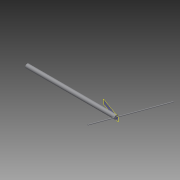
# Autodesk Inventor part: Piston_Model
Saved by Autodesk Inventor 2015 (Build 190159000, 159)
## iProperties
Created: 2017-01-24
Part Number: Piston_Model
Material: Generic
Document SubType Name: Modeling
Designer: Guy
Density: 1 g/cm^3
Appearance: Default
Author: Guy
Autodesk Inventor part; units mm, degrees
ref_plane "YZ Plane" through (0, 0, 0) normal (1, 0, 0) x (0, 1, 0)
ref_plane "XZ Plane" through (0, 0, 0) normal (0, 1, 0) x (-1, 0, 0)
ref_plane "XY Plane" through (0, 0, 0) normal (0, 0, 1) x (1, 0, 0)
sketch "Sketch1" plane through (0, 0, 0) normal (1, 0, 0) x (0, 1, 0)
  circle A0 centre (0, 0) radius 4.435
  dimension "d0" = 8.87
  constraints: 1 centre point, 1 coincident
  measures "d0" diameter of A0
extrude "Extrusion1" add sketch "Sketch1" along normal blind 200
sketch "Sketch2" plane through (200, 0, 0) normal (1, 0, 0) x (0, 0, -1)
  circle A0 centre (0, 0) radius 4.435 projected
  line L0 (0, 0) -> (8.3226, 0)
  line L1 (0.8914, 0) -> (-7.5966, 0)
  arc A1 (-4.435, 0) -> (4.435, 0) centre (0, 0) ccw
  constraints: 4 end point, 3 point on line, 2 horizontal, 2 point on circle, 1 centre point, 1 coincident, 1 concentric
extrude "Extrusion2" add sketch "Sketch2" along normal blind 0.01 contours A0 L1 L0 picked at (-2.4155, -1.6673)
ref_plane "Work Plane1" through (200.01, 0, 0) normal (0.3420201, 0.9396926, 0) x (0, 0, 1)
sketch "Sketch4" plane through (200.01, 0, 0) normal (0.3420201, 0.9396926, 0) x (0, 0, 1)
  line L0 (4.435, -0.0094) -> (-4.435, -0.0094) projected
  ellipse E0 centre (0, -0.0094) end of major axis (-4.435, -0.0094) minor radius 1.5169 (-4.435, -0.0094) -> (4.435, -0.0094) ccw projected
  line L1 (-4.435, 0) -> (4.435, 0) projected
  ellipse E1 centre (0, 0) end of major axis (-4.435, 0) minor radius 1.5169 (4.435, 0) -> (-4.435, 0) ccw projected
  circle A0 centre (0, 0) radius 1
  point P0 (0, -187.9479)
  dimension "d11" = 2
  constraints: 1 centre point, 1 coincident, 2 other
  measures "d11" diameter of A0
extrude "Extrusion4" add sketch "Sketch4" along normal blind 100 and the other way blind 50 contours A0 L0 | L0 A0 L1 | L1 A0
body "Solid1"
